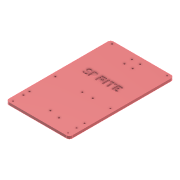
# Autodesk Inventor part: top plate
Saved by Autodesk Inventor 2022 (Build 260153000, 153)
## iProperties
Created: 2024-03-20
Part Number: top plate
Material: Generic
Document SubType Name: Modeling
Designer: david
Density: 1 g/cm^3
Appearance: Smooth - Red
Author: david
Autodesk Inventor part; units mm, degrees
ref_plane "YZ Plane" through (0, 0, 0) normal (1, 0, 0) x (0, 1, 0)
ref_plane "XZ Plane" through (0, 0, 0) normal (0, 1, 0) x (-1, 0, 0)
ref_plane "XY Plane" through (0, 0, 0) normal (0, 0, 1) x (1, 0, 0)
sketch "Sketch1" plane through (0, 0, 0) normal (0, 1, 0) x (-1, 0, 0)
  line L0 (57.5, -190) -> (57.5, -190) construction
  line L1 (-57.5, -190) -> (-57.5, 0) construction
  line L2 (-57.5, 0) -> (57.5, 0)
  line L3 (57.5, 0) -> (57.5, -190) construction
  line L4 (80.5, 0) -> (-80.5, 0) construction
  line L5 (0, -228) -> (0, 38) construction
  line L6 (57.5, -190) -> (-57.5, -190)
  line L7 (-57.5, -190) -> (-57.5, -190) construction
  line L8 (57.5, 0) -> (-55.1767, 0)
  line L9 (57.5, -40) -> (-57.5, -40) construction
  line L10 (-57.5, -40) -> (-57.5, 0)
  line L11 (-57.5, 0) -> (57.5, 0)
  line L12 (57.5, 0) -> (57.5, -40)
  line L13 (-57.5, -190) -> (-57.5, -40)
  line L14 (57.5, -190) -> (57.5, -40)
  point P0 (0, 0)
  dimension "width" = 115
  dimension "Length" = 190
  dimension "d2" = 115
  dimension "d112" = 40
  constraints: 26 end point, 6 parallel, 5 horizontal, 4 perpendicular, 1 collinear, 1 point on line, 1 symmetric about line, 1 vertical alignment, 1 other
  measures "width" distance of L1.end L2.end
  measures "Length" distance of L1.start L1.end
  measures "d2" distance of L6.end L0.end
  measures "d112" distance between parallel lines of L2 L9
extrude "Base" add sketch "Sketch1" against normal blind 5
sketch "Sketch11" plane through (0, 0, 0) normal (0, 1, 0) x (1, 0, 0)
  line L0 (0, 228) -> (0, -38) construction
  line L1 (-57.5, 0) -> (57.5, 0) construction
  line L2 (57.5, 190) -> (-57.5, 190) projected
  line L3 (-50, 5) -> (50, 5) construction
  line L4 (50, 5) -> (50, 35) construction
  line L5 (50, 35) -> (-50, 35) construction
  line L6 (-50, 35) -> (-50, 5) construction
  point P0 (0, 0)
  point P1 (50, 185)
  point P2 (-50, 185)
  dimension "d91" = 5
  dimension "d92" = 50
  dimension "d93" = 5
  dimension "d94" = 50
  dimension "d113" = 30
  constraints: 8 end point, 2 coincident, 2 parallel, 2 symmetric about line, 1 horizontal, 1 perpendicular, 1 vertical alignment
  measures "d91" distance from line of L1 point (50, 5)
  measures "d92" distance from line of point (50, 5) L0
  measures "d93" distance from line of L2 point (50, 185)
  measures "d94" distance from line of L0 point (50, 185)
  measures "d113" distance of L3.end L4.end
hole "Mounting Holes" at (50, 0, -5) at (-50, 0, -5) at (50, 0, -185) at (-50, 0, -185) at (-50, 0, -35) at (50, 0, -35) direction (0, -1, 0) diameter 3.4 depth 6
fillet "Fillet1" radius 5 4 edges at (-57.5, -2.5, 0) (57.5, -2.5, -190) (-57.5, -2.5, -190) (57.5, -2.5, 0)
sketch "Sketch12" plane through (0, 0, 0) normal (0, 1, 0) x (1, 0, 0)
  line L0 (-50, 82) -> (-1, 82) construction
  line L1 (-1, 82) -> (-1, 24) construction
  line L2 (-1, 24) -> (-50, 24) construction
  line L3 (-50, 24) -> (-50, 82) construction
  line L4 (-57.5, 185) -> (-57.5, 5) projected
  line L5 (0, 228) -> (0, -38) projected
  line L6 (-52.5, 0) -> (52.5, 0) projected
  circle A0 centre (-50, 35) radius 1.7 projected
  point P0 (0, 0)
  point P1 (0, 0)
  point P2 (52.2987, 0)
  point P3 (-57.5, 40)
  point P4 (0, 0)
  dimension "d103" = 49
  dimension "d104" = 58
  dimension "d239" = 24
  constraints: 8 end point, 2 parallel, 1 horizontal, 1 midpoint, 1 perpendicular, 1 vertical alignment
  measures "d103" distance of L1.end L2.end
  measures "d104" distance of L0.end L1.end
  measures "d239" distance between parallel lines of L6 L2
hole "RasPi Mounting Holes" at (-50, 0, -82) at (-1, 0, -82) at (-1, 0, -24) at (-50, 0, -24) direction (0, -1, 0) diameter 3.4 depth 6
sketch "Sketch15" plane through (0, 0, 0) normal (0, 1, 0) x (1, 0, 0)
  line L0 (50, 82) -> (50, 20.5) construction
  line L1 (50, 20.5) -> (18, 20.5) construction
  line L2 (18, 20.5) -> (18, 82) construction
  line L3 (18, 82) -> (50, 82) construction
  line L4 (-52.5, 0) -> (52.5, 0) projected
  circle A0 centre (-1, 82) radius 1.7 projected
  circle A1 centre (50, 35) radius 1.7 projected
  point P0 (0, 0)
  point P1 (0, 0)
  dimension "d122" = 32
  dimension "d123" = 61.5
  constraints: 8 end point, 4 coincident, 2 parallel, 1 horizontal alignment, 1 midpoint, 1 perpendicular, 1 vertical, 1 vertical alignment
  measures "d122" distance of L2.end L0.start
  measures "d123" distance of L1.end L2.end
hole "LM2596 Mounting Holes" at (50, 0, -82) at (50, 0, -20.5) at (18, 0, -20.5) at (18, 0, -82) direction (0, -1, 0) diameter 3.4 depth 6
sketch "Sketch16" plane through (0, 0, 0) normal (0, 1, 0) x (1, 0, 0)
  line L0 (-7.5, 165) -> (7.5, 165) construction
  line L1 (7.5, 165) -> (7.5, 178.5) construction
  line L2 (7.5, 178.5) -> (-7.5, 178.5) construction
  line L3 (-7.5, 178.5) -> (-7.5, 165) construction
  line L4 (52.5, 190) -> (-52.5, 190) projected
  point P0 (0, 0)
  point P1 (0, 178.5)
  point P2 (0, 190)
  dimension "d132" = 15
  dimension "d133" = 13.5
  dimension "d251" = 11.5
  constraints: 8 end point, 4 coincident, 2 midpoint, 2 parallel, 1 horizontal, 1 perpendicular, 1 vertical alignment
  measures "d132" distance of L1.end L2.end
  measures "d133" distance of L2.end L0.start
  measures "d251" distance between parallel lines of L2 L4
hole "Camera Mount Mounting Holes" at (-7.5, 0, -178.5) at (-7.5, 0, -165) at (7.5, 0, -165) at (7.5, 0, -178.5) direction (0, -1, 0) diameter 3.4 depth 6
sketch "Sketch17" plane through (0, 0, 0) normal (0, 1, 0) x (1, 0, 0)
  line L0 (-57.1973, 19.3379) -> (-57.1973, 79.4802) construction
  line L1 (-57.1973, 79.4802) -> (-14.6793, 79.4802) construction
  line L2 (-14.6793, 79.4802) -> (-14.6793, 19.3379) construction
  line L3 (-14.6793, 19.3379) -> (-57.1973, 19.3379) construction
  circle A0 centre (-50, 24) radius 1.7 projected
  circle A1 centre (-50, 82) radius 1.7 projected
  line L4 (-52.5, 0) -> (52.5, 0) projected
  spline S0 degree 4 poles (-24.5389, 124.9198) (-24.922, 125.4965) (-27.6826, 126.8954) (-30.1628, 126.7912) (-32.1332, 125.7629) (-33.4299, 124.0907) (-33.6545, 122.2258) (-32.7478, 119.1755) (-29.7631, 118.647) (-24.9617, 117.5574) (-28.1153, 114.1457) (-30.627, 115.8823) (-32.3688, 117.1404) knots 0 0 0 0 0 0.20272 0.281354 0.3552 0.433005 0.51958 0.610323 0.697239 0.780233 1 1 1 1 1
  line L5 (-32.3688, 117.1404) -> (-33.9542, 115.1175)
  line L6 (-24.5389, 124.9198) -> (-25.9227, 122.7407)
  spline S1 degree 4 poles (-25.9227, 122.7407) (-26.5371, 123.0059) (-27.0432, 123.8303) (-29.8104, 124.5696) (-31.1048, 122.982) (-30.4927, 121.5853) (-28.2889, 121.2516) (-27.5721, 120.9152) (-25.6358, 120.2756) (-24.5434, 118.9786) (-23.9735, 117.8945) (-24.2985, 114.6128) (-27.371, 112.453) (-32.008, 112.9595) (-33.5375, 114.8946) (-33.9542, 115.1175) knots 0 0 0 0 0 0.144957 0.205265 0.266901 0.324627 0.385746 0.449034 0.509011 0.57578 0.647336 0.72838 0.816759 1 1 1 1 1
  line L7 (-23.2822, 126.3237) -> (-23.2822, 113.2811)
  line L8 (-23.2822, 113.2811) -> (-20.5533, 113.2884)
  line L9 (-20.5533, 113.2884) -> (-20.5533, 117.1404)
  line L10 (-20.5436, 123.784) -> (-20.5436, 119.7226)
  line L11 (-20.5436, 119.7226) -> (-18.2264, 119.7226)
  line L12 (-20.5436, 123.784) -> (-18.2264, 123.784)
  line L13 (-23.2822, 126.3237) -> (-18.1485, 126.3237)
  line L14 (-20.5533, 117.1404) -> (-18.1485, 117.1404)
  spline S2 degree 4 poles (-18.1485, 126.3237) (-16.6845, 126.5227) (-13.988, 125.7234) (-13.1568, 120.9814) (-14.2131, 118.7079) (-16.0401, 117.1114) (-18.1485, 117.1404) knots 0 0 0 0 0 0.42308 0.582818 1 1 1 1 1
  spline S3 degree 4 poles (-18.2264, 123.784) (-16.7633, 123.9916) (-15.1954, 121.9939) (-16.394, 119.8116) (-18.2264, 119.7226) knots 0 0 0 0 0 1 1 1 1 1
  line L15 (-9.8541, 122.5443) -> (-9.8541, 113.2671)
  line L16 (-9.8541, 113.2671) -> (-6.5382, 113.2671)
  line L17 (-6.5382, 113.2671) -> (-6.5382, 113.4426)
  line L18 (-6.5382, 113.4426) -> (-6.5382, 117.1888)
  line L19 (-6.5382, 117.1888) -> (-4.8269, 117.1888)
  line L20 (-4.8269, 117.1888) -> (-2.3071, 113.2671)
  line L21 (-2.3071, 113.2671) -> (1.6946, 113.2671)
  line L22 (1.6946, 113.2671) -> (-0.8253, 117.1888)
  line L23 (-9.8541, 122.5443) -> (-6.5382, 122.5443)
  line L24 (-6.5382, 122.5443) -> (-6.5382, 120.5743)
  line L25 (-6.5382, 120.5743) -> (-2.6026, 120.5743)
  line L26 (-2.6026, 120.5743) -> (-2.6026, 123.1634)
  line L27 (-2.6026, 123.1634) -> (-9.8541, 123.1634)
  line L28 (-9.8541, 123.1634) -> (-9.8541, 126.4713)
  line L29 (-9.8541, 126.4713) -> (-0.5373, 126.4713)
  line L30 (0.769, 125.022) -> (0.769, 118.8518)
  arc A2 (-0.8253, 117.1888) -> (0.769, 118.8518) centre (-0.9621, 118.9157) ccw
  arc A3 (0.769, 125.022) -> (-0.5373, 126.4713) centre (-1.5712, 124.2261) ccw
  line L31 (2.6608, 126.4713) -> (6.0256, 126.4713)
  line L32 (6.0256, 126.4713) -> (6.0256, 113.2671)
  line L33 (6.0256, 113.2671) -> (2.6608, 113.2671)
  line L34 (2.6608, 113.2671) -> (2.6608, 126.4713)
  line L35 (7.5596, 126.4713) -> (7.5596, 123.1634)
  line L36 (7.5596, 123.1634) -> (10.9283, 123.1634)
  line L37 (10.9283, 123.1634) -> (10.9283, 113.2671)
  line L38 (10.9283, 113.2671) -> (14.2393, 113.2671)
  line L39 (14.2393, 113.2671) -> (14.2393, 126.4713)
  line L40 (14.2393, 126.4713) -> (7.5596, 126.4713)
  line L41 (14.8531, 126.4713) -> (14.8531, 123.1634)
  line L42 (14.8531, 123.1634) -> (17.2975, 123.1634)
  line L43 (17.2975, 123.1634) -> (19.544, 126.4713)
  line L44 (19.544, 126.4713) -> (14.8531, 126.4713)
  line L45 (20.2187, 126.4775) -> (20.2187, 113.2671)
  line L46 (20.2187, 113.2671) -> (23.5406, 113.2671)
  line L47 (23.5406, 113.2671) -> (23.5406, 126.4775)
  line L48 (23.5406, 126.4775) -> (20.2187, 126.4775)
  line L49 (24.1159, 121.5593) -> (24.1159, 118.2075)
  line L50 (24.1159, 118.2075) -> (26.608, 118.2075)
  line L51 (26.608, 118.2075) -> (26.608, 121.5593)
  line L52 (26.608, 121.5593) -> (24.1159, 121.5593)
  line L53 (23.5406, 126.4775) -> (23.5406, 123.1396)
  line L54 (23.5406, 123.1396) -> (28.6492, 123.1396)
  line L55 (28.6492, 123.1396) -> (28.6492, 126.4775)
  line L56 (28.6492, 126.4775) -> (23.5406, 126.4775)
  line L57 (28.6492, 126.4775) -> (30.8175, 123.1396)
  line L58 (30.8175, 123.1396) -> (28.6492, 123.1396)
  line L59 (26.608, 121.5593) -> (28.8205, 121.5315)
  line L60 (28.8205, 121.5315) -> (26.608, 118.2075)
  line L61 (23.5406, 116.6064) -> (30.8177, 116.6064)
  line L62 (30.8177, 116.6064) -> (28.6492, 113.2671)
  line L63 (28.6492, 113.2671) -> (23.5406, 113.2671)
  line L64 (-20.5533, 113.2884) -> (-7.3915, 113.2884)
  line L65 (-57.5, 185) -> (-57.5, 5) projected
  line L66 (57.5, 5) -> (57.5, 185) projected
  line L67 (57.5, 185) -> (57.5, 5) projected
  point P0 (0, 0)
  point P1 (-35.9383, 19.3379)
  point P2 (0, 0)
  point P3 (-26.0743, 125.9223)
  point P4 (-28.9193, 126.6257)
  point P5 (-32.067, 125.6116)
  point P6 (-33.4554, 122.3675)
  point P7 (-29.2911, 118.5075)
  point P8 (-26.9401, 117.3059)
  point P9 (-27.1681, 116.1283)
  point P10 (-28.939, 115.4933)
  point P11 (-32.4456, 119.8309)
  point P12 (-33.1379, 124.2152)
  point P13 (-30.7742, 126.3572)
  point P14 (-26.7112, 123.2461)
  point P15 (-28.1768, 123.919)
  point P16 (-30.0893, 123.8265)
  point P17 (-30.7803, 122.924)
  point P18 (-30.2965, 121.8845)
  point P19 (-28.5195, 121.2364)
  point P20 (-27.4225, 120.886)
  point P21 (-25.8005, 120.143)
  point P22 (-24.69, 119.0688)
  point P23 (-24.2101, 117.9282)
  point P24 (-24.53, 115.3475)
  point P25 (-26.7119, 113.3702)
  point P26 (-30.6972, 113.2718)
  point P27 (-33.2613, 114.5685)
  point P28 (-15.6674, 125.8448)
  point P29 (-14.0095, 123.9105)
  point P30 (-13.6514, 121.4185)
  point P31 (-14.0618, 119.634)
  point P32 (-15.2337, 118.127)
  point P33 (-16.9529, 123.3565)
  point P34 (-16.2765, 122.0378)
  point P35 (-16.6728, 120.5472)
  point P36 (0, 106.588)
  constraints: 120 end point, 8 point on line, 4 point on circle, 2 centre point, 2 midpoint, 2 vertical, 1 horizontal, 50 other
extrude "SP RITE" cut sketch "Sketch17" against normal blind 2 contours L6 S1 L5 S0 | L13 S2 L14 L9 L8 L7 | L15 L23 L24 L25 L26 L27 L28 L29 A3 L30 A2 L22 L21 L20 L19 L18 L17 L16 | L12 S3 L11 L10 | L31 L32 L33 L34 | L40 L39 L38 L37 L36 L35 | L44 L43 L42 L41 | L48 L47 L46 L45 | L56 L55 L54 L47 | L47 L61 L62 L63 | L57 L58 L55 | L52 L51 L50 L49 | L59 L60 L51
equation "\"d2\" = width"
equation "\"d93\" = d91"
equation "\"d94\" = d92"
equation "\"d95\" = HoleDia"
equation "\"d105\" = HoleDia"
equation "\"d125\" = HoleDia"
equation "\"d135\" = HoleDia"
equation "\"HoleDia\" = 3.4"
body "Solid1"
